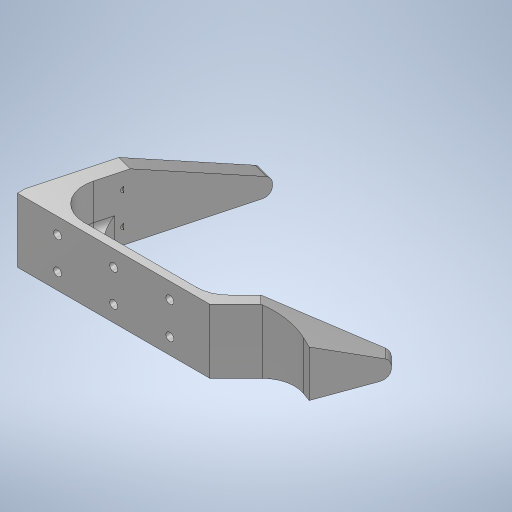
# Autodesk Inventor part: Forks
Saved by Autodesk Inventor 2023.4 (Build 274418000, 418)
## iProperties
Created: 2024-05-15
Part Number: Forks
Material: UHMW, White
Document SubType Name: Modeling
Designer: Nathan Cai
Density: 0.94 g/cm^3
Appearance: Rubber - Black - Version 1.1
Author: Nathan Cai
Autodesk Inventor part; units mm, degrees
ref_plane "YZ Plane" through (0, 0, 0) normal (1, 0, 0) x (0, 1, 0)
ref_plane "XZ Plane" through (0, 0, 0) normal (0, 1, 0) x (-1, 0, 0)
ref_plane "XY Plane" through (0, 0, 0) normal (0, 0, 1) x (1, 0, 0)
sketch "Sketch1" plane through (0, 0, 0) normal (0, 0, 1) x (1, 0, 0)
  line L0 (-38.1, -12.7) -> (38.1, -12.7)
  line L1 (38.1, -12.7) -> (38.1, 12.7)
  line L2 (38.1, 12.7) -> (-38.1, 12.7)
  line L3 (-38.1, 12.7) -> (-38.1, -12.7)
  line L4 (-38.1, -12.7) -> (38.1, 12.7) construction
  line L5 (38.1, -12.7) -> (-38.1, 12.7) construction
  circle A0 centre (-22.225, 6.35) radius 1.5 construction
  point P0 (0, 0)
  point P1 (0, 6.35)
  point P2 (22.225, 6.35)
  point P3 (-22.225, -6.35)
  point P4 (0, -6.35)
  point P5 (22.225, -6.35)
  dimension "d0" = 76.2
  dimension "d1" = 25.4
  dimension "d2" = 3
  dimension "d3" = 6.35
  dimension "d4" = 22.225
  dimension "d7" = 22.225
  dimension "d10" = 12.7
  constraints: 12 end point, 2 horizontal, 2 midpoint, 2 parallel, 1 centre point, 1 coincident, 1 perpendicular, 1 vertical, 5 other
  measures "d0" distance of L2.end L1.end
  measures "d1" distance of L1.end L0.end
  measures "d2" diameter of A0
  measures "d3" vertical distance of point (0, 0) A0.centre
  measures "d4" horizontal distance of point (0, 0) A0.centre
  measures "d7" distance of point (-22.225, 6.35) point (0, 6.35)
  measures "d10" distance of point (-22.225, 6.35) point (-22.225, -6.35)
extrude "Extrusion1" add sketch "Sketch1" along normal blind 3.175
sketch "Sketch2" plane through (-38.1, 12.7, 0) normal (0, 1, 0) x (1, 0, 0)
  line L0 (76.2, -3.175) -> (112.121024, 32.746024)
  line L1 (112.121024, 32.746024) -> (108.946024, 35.921024)
  line L2 (108.946024, 35.921024) -> (73.025, 0)
  line L3 (73.025, 0) -> (76.2, -3.175)
  line L4 (76.2, -3.175) -> (127, -3.175) construction
  line L5 (76.2, 0) -> (0, 0)
  line L6 (0, 0) -> (19.722011, 73.603548)
  line L7 (19.722011, 73.603548) -> (25.85564, 71.960047)
  line L8 (25.85564, 71.960047) -> (6.133629, -1.643501)
  line L9 (6.133629, -1.643501) -> (0, 0)
  line L10 (0, 0) -> (76.2, 0) construction
  line L11 (112.121024, 32.746024) -> (103.433713, 8.877832)
  line L12 (103.433713, 8.877832) -> (92.303792, 12.928792)
  point P0 (38.1, 0)
  point P1 (6.574004, 0)
  dimension "d15" = 50.8
  dimension "d16" = 45
  dimension "d17" = 76.2
  dimension "d18" = 75
  dimension "d19" = 6.35
  dimension "d48" = 25
  dimension "d49" = 25.4
  constraints: 24 end point, 4 parallel, 3 perpendicular, 2 equal length, 2 horizontal, 2 point on line
  measures "d15" distance of L0.start L0.end
  measures "d16" angle of L4 L0
  measures "d17" distance of L5.end L6.end
  measures "d18" angle of L10 L6
  measures "d19" distance of L6.end L7.end
  measures "d48" angle of L0 L11
  measures "d49" distance from line of L0.end L12
extrude "Extrusion2" add sketch "Sketch2" against normal up to surface (25.4 mm away) contours L3 L2 L1 L0 | L0 L11 L12 | L5 L6 L7 L8
fillet "Fillet1" radius 12.7 3 edges at (-31.526, 0, 0) (34.925, 0, 0) (54.2038, 0, -12.9288)
chamfer "Chamfer1" distance 36.5125 distance2 19.05 1 edges at (72.4335, 12.7, -34.3335) measured on face at (72.08, 12.7, -33.98)
chamfer "Chamfer2" distance 46.0375 distance2 19.05 1 edges at (-15.3112, 12.7, -72.7818) measured on face at (-15.4406, 12.7, -72.2988)
fillet "Fillet2" radius 3.175 4 edges at (72.4335, -6.35, -34.3335) (72.4335, -12.7, -34.3335) (-15.3112, -6.35, -72.7818) (-15.3112, -12.7, -72.7818)
sketch "Sketch4" plane through (-38.1, -12.7, 3.175) normal (0, -1, 0) x (1, 0, 0)
  line L0 (25.03389, -72.068233) -> (18.900261, -73.711733)
  line L1 (10.857708, -19.162002) -> (25.03389, -72.068233)
  arc A0 (23.124966, -3.175) -> (10.857708, -19.162002) centre (23.124966, -15.875) ccw
  line L2 (23.124966, -3.175) -> (67.764488, -3.175)
  arc A1 (76.744744, -6.894744) -> (67.764488, -3.175) centre (67.764488, -15.875) ccw
  line L3 (106.70096, -36.85096) -> (76.744744, -6.894744)
  line L4 (110.922851, -32.62907) -> (106.70096, -36.85096)
  line L5 (76.2, 0) -> (86.582738, -10.382738)
  line L6 (0, 0) -> (76.2, 0)
  line L7 (0, -3.175) -> (0, 0)
  line L8 (18.900261, -73.711733) -> (0, -3.175)
  arc A2 (23.124966, -3.175) -> (10.857708, -19.162002) centre (23.124966, -15.875) ccw
  line L9 (83.127788, -13.277788) -> (76.744744, -6.894744)
  line L10 (10.857708, -19.162002) -> (76.744744, -6.894744)
  line L11 (103.433713, -12.052832) -> (110.922851, -32.62907)
  line L12 (99.90665, -13.336578) -> (103.433713, -12.052832)
  arc A3 (86.582738, -10.382738) -> (99.90665, -13.336578) centre (95.562994, -1.402482) ccw
  point P0 (38.1, -3.175)
  constraints: 2 end point
extrude "Extrusion3" add sketch "Sketch4" against normal blind 4.7625 contours A0 L2 A1 L10
fillet "Fillet3" radius 6.35 2 edges at (38.6447, -10.3187, -3.7197) (-27.2423, -10.3187, -15.987)
fillet "Fillet4" radius 6.35 5 edges at (-26.3541, -7.9375, -19.3019) (7.3447, -7.9375, 0) (34.5246, -7.9375, -0.9667) (39.8271, -7.9375, -4.9021) (-25.0506, -7.9375, -4.9687)
hole "Hole1" at (-22.225, 6.35, 0) at (0, 6.35, 0) at (22.225, 6.35, 0) at (-22.225, -6.35, 0) at (0, -6.35, 0) at (22.225, -6.35, 0) direction (0, 0, 1) diameter 3.2004 end through all clearance for "Socket Head Cap Screw" size "M3" standard "Ansi Metric M Profile"
hole "Hole2" at (-22.225, 6.35, 0) at (0, 6.35, 0) at (22.225, 6.35, 0) at (22.225, -6.35, 0) at (0, -6.35, 0) at (-22.225, -6.35, 0) direction (0, 0, -1) diameter 5.5 depth 25.4
equation "\"d7\" = d4"
equation "\"d10\" = 2 * d3"
body "Solid1"
